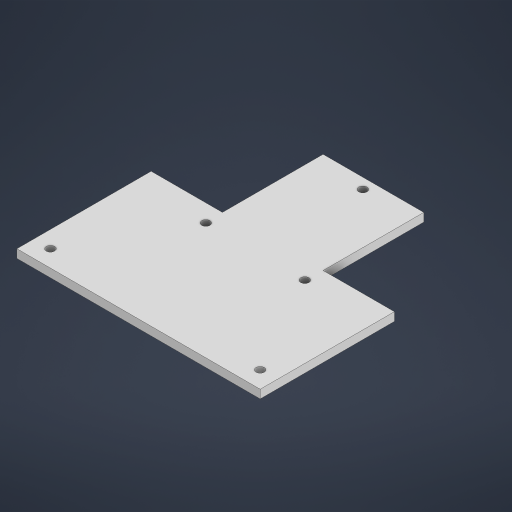
# Autodesk Inventor part: chasis_tapa
Saved by Autodesk Inventor 2023 (Build 270158000, 158)
## iProperties
Created: 2022-08-22
Part Number: chasis_tapa
Material: Generic
Document SubType Name: Modeling
Designer: marat
Density: 1 g/cm^3
Appearance: Default
Author: marat
Autodesk Inventor part; units mm, degrees
ref_plane "YZ Plane" through (0, 0, 0) normal (1, 0, 0) x (0, 1, 0)
ref_plane "XZ Plane" through (0, 0, 0) normal (0, 1, 0) x (-1, 0, 0)
ref_plane "XY Plane" through (0, 0, 0) normal (0, 0, 1) x (1, 0, 0)
sketch "Sketch1" plane through (0, 0, 0) normal (0, 1, 0) x (-1, 0, 0)
  line L0 (72.5, 40) -> (-72.5, 40)
  line L1 (-72.5, 40) -> (-72.5, -40)
  line L2 (-72.5, -40) -> (72.5, -40)
  line L3 (72.5, -40) -> (72.5, 40)
  line L4 (72.5, 40) -> (-72.5, -40) construction
  line L5 (-72.5, 40) -> (72.5, -40) construction
  line L6 (30, -40) -> (-30, -40)
  line L7 (-30, -40) -> (-30, -100)
  line L8 (-30, -100) -> (30, -100)
  line L9 (30, -100) -> (30, -40)
  point P0 (0, 0)
  dimension "d0" = 145
  dimension "d1" = 80
  dimension "d2" = 60
  dimension "d3" = 60
  dimension "d4" = 42.5
  constraints: 20 end point, 4 parallel, 2 midpoint, 2 perpendicular, 2 point on line, 1 horizontal
  measures "d0" distance of L2.end L1.end
  measures "d1" distance of L1.end L0.end
  measures "d2" distance of L7.end L6.end
  measures "d3" distance between parallel lines of L7 L9
  measures "d4" distance between parallel lines of L3 L9
extrude "Extrusion1" add sketch "Sketch1" along normal blind 5
sketch "Sketch2" plane through (0, 5, 0) normal (0, 1, 0) x (1, 0, 0)
  circle A0 centre (62.5, -30.0138) radius 2.5
  circle A1 centre (-29.5, 29.592) radius 2.5
  circle A2 centre (-62.5, -30) radius 2.5
  circle A3 centre (29.5, 29.6088) radius 2.5
  line L0 (-72.5, 25.8201) -> (-72.5, -40)
  line L1 (-72.5, -40) -> (79.2535, -40)
  circle A4 centre (0, 93.693) radius 2.5
  line L2 (-72.5, -40) -> (72.5, -40) projected
  line L3 (-72.5, 40) -> (-72.5, -40) projected
  point P0 (0, 0)
  point P1 (0, 0)
  dimension "d1" = 80
  dimension "d7" = 5
  dimension "d8" = 5
  dimension "d9" = 5
  dimension "d10" = 5
  dimension "d11" = 59
  dimension "d12" = 125
  dimension "d13" = 33
  dimension "d14" = 59.592
  dimension "d15" = 10
  dimension "d16" = 10
  dimension "d17" = 5
  dimension "d18" = 64.101
  dimension "d19" = 0
  dimension "d20" = 0
  constraints: 5 centre point, 4 end point
  measures "d7" diameter of A0
  measures "d8" diameter of A2
  measures "d9" diameter of A1
  measures "d10" diameter of A3
  measures "d11" distance of A3.centre A1.centre
  measures "d12" distance of A0.centre A2.centre
  measures "d13" horizontal distance of A1.centre A2.centre
  measures "d14" vertical distance of A2.centre A1.centre
  measures "d15" distance from line of L0 A2.centre
  measures "d16" distance from line of L1 A2.centre
  measures "d17" diameter of A4
  measures "d18" vertical distance of A4.centre A1.centre
  measures "d19" distance between parallel lines of L2 L1
  measures "d20" distance between parallel lines of L3 L0
extrude "Extrusion2" cut sketch "Sketch2" against normal through all
body "Solid1"
